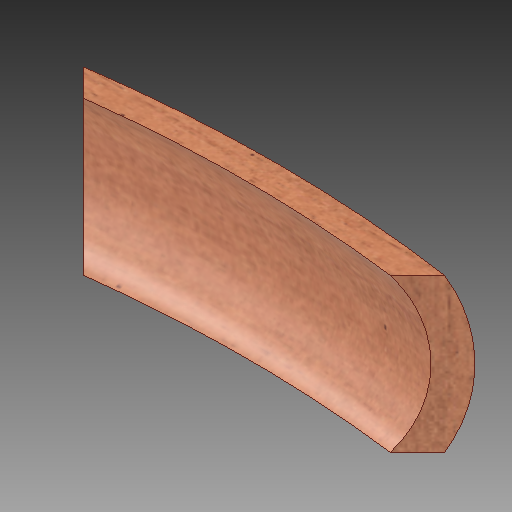
# Autodesk Inventor part: dou_long
Saved by Autodesk Inventor 2019 (Build 230136000, 136)
## iProperties
Created: 2019-11-15
Part Number: dou_long
Material: Красное дерево
Document SubType Name: Modeling
Designer: stepa
Density: 0.512 g/cm^3
Appearance: Красное дерево — натуральный — полированный
Mass: 106.218 g
Surface Area: 396.549 cm^2
Volume: 207.457 cm^3
Author: stepa
Autodesk Inventor part; units mm, degrees
ref_plane "YZ Plane" through (0, 0, 0) normal (1, 0, 0) x (0, 1, 0)
ref_plane "XZ Plane" through (0, 0, 0) normal (0, 1, 0) x (-1, 0, 0)
ref_plane "XY Plane" through (0, 0, 0) normal (0, 0, 1) x (1, 0, 0)
sketch "Эскиз1" plane through (0, 0, 0) normal (0, 1, 0) x (-1, 0, 0)
  line L0 (0, 0) -> (-220, 0)
  line L1 (-220, 0) -> (-220, -30)
  line L2 (-220, -30) -> (0, -30)
  line L3 (0, -30) -> (0, 0)
  dimension "d0" = 220
  dimension "d1" = 30
  constraints: 8 end point, 2 parallel, 1 horizontal, 1 perpendicular
  measures "d0" distance of L2.end L1.end
  measures "d1" distance of L1.end L0.end
extrude "Выдавливание1" add sketch "Эскиз1" along normal blind 80
chamfer "Фаска1" distance 30 angle 45 2 edges at (0, 40, 0) (220, 40, 0)
sketch "Эскиз2" plane through (0, 80, 0) normal (0, 1, 0) x (1, 0, 0)
  line L0 (220, 30) -> (190, 0) projected
  line L1 (220, 30) -> (0, 30) projected
  line L2 (30, 0) -> (0, 30) projected
  line L3 (30, 0) -> (190, 0) projected
  arc A0 (212.0711, 22.0711) -> (7.9289, 22.0711) centre (110, -630.9573) ccw
  line L4 (0, 30) -> (30, 0) projected
  line L5 (15, 15) -> (7.9289, 22.0711)
  line L6 (220, 30) -> (190, 0) projected
  line L7 (220, 30) -> (0, 30) projected
  arc A1 (190, 0) -> (30, 0) centre (110, -630.9573) ccw
  line L8 (30, 0) -> (190, 0) projected
  point P0 (0, 0)
  point P1 (110, 0)
  point P2 (110, 0)
  dimension "d7" = 10
  constraints: 4 point on circle, 4 point on line, 3 midpoint, 2 centre point, 2 end point, 2 horizontal alignment, 2 vertical alignment, 1 concentric, 1 tangent
  measures "d7" distance of L5.start L5.end
extrude "Выдавливание2" cut sketch "Эскиз2" against normal through all contours L0 A0 L1 | A0 L2 L1 | L3 A1
sketch "Эскиз3" plane through (212.0711, 0, -22.0711) normal (0.7071068, 0, 0.7071068) x (0.7071068, 0, -0.7071068)
  line L0 (0, 0) -> (0, 80) projected
  line L1 (0, 80) -> (-31.2132, 80) projected
  line L2 (-31.2132, 80) -> (-31.2132, 0) projected
  line L3 (-31.2132, 0) -> (0, 0) projected
  line L4 (0, 80) -> (-31.2132, 80) projected
  arc A0 (-11.2132, 0) -> (-11.2132, 80) centre (-76.9511, 40) ccw
  line L5 (-31.2132, 0) -> (0, 0) projected
  line L6 (0, 0) -> (0, 80) projected
  arc A1 (-31.2132, 0) -> (-31.2132, 80) centre (-76.9511, 40) ccw
  line L7 (-31.2132, 80) -> (-31.2132, 0) projected
  line L8 (-31.2132, 0) -> (-11.2132, 0)
  line L9 (-31.2132, 80) -> (-11.2132, 80)
  point P0 (-31.2132, 40)
  point P1 (-31.2132, 40)
  dimension "d10" = 20
  dimension "d11" = 60.7614
  dimension "d12" = 76.9511
  constraints: 4 end point, 4 point on circle, 2 centre point, 2 collinear, 2 horizontal alignment, 2 midpoint, 2 point on line, 1 concentric, 1 tangent
  measures "d10" distance of L1.end L9.end
  measures "d11" radius of A1
  measures "d12" radius of A0
sketch3d "3D эскиз1"
  arc A0 (212.0711, 80, -22.0711) -> (7.9289, 80, -22.0711) centre (110, 80, 630.9573) ccw
sweep "Сдвиг1" cut profiles "Эскиз3" path "3D эскиз1" contours L3 A0 L0 | A0 L1 L0 | L2 A1
